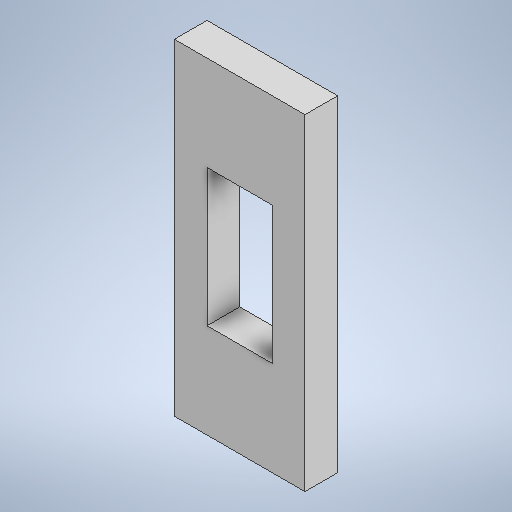
# Autodesk Inventor part: placa de amarre
Saved by Autodesk Inventor 2025.2 (Build 292293000, 293)
## iProperties
Created: 2025-03-06
Part Number: placa de amarre
Material: Genérico
Document SubType Name: Modeling
Designer: julia
Density: 1 g/cm^3
Appearance: Valor por defecto
Author: julia
Autodesk Inventor part; units mm, degrees
ref_plane "YZ Plane" through (0, 0, 0) normal (1, 0, 0) x (0, 1, 0)
ref_plane "XZ Plane" through (0, 0, 0) normal (0, 1, 0) x (-1, 0, 0)
ref_plane "XY Plane" through (0, 0, 0) normal (0, 0, 1) x (1, 0, 0)
sketch "Boceto1" plane through (0, 0, 0) normal (0, 0, 1) x (1, 0, 0)
  line L0 (0, 0) -> (2, 0)
  line L1 (2, 0) -> (2, 5)
  line L2 (2, 5) -> (0, 5)
  line L3 (0, 5) -> (0, 0)
  line L4 (0.5, 1.45) -> (1.5, 1.45)
  line L5 (1.5, 1.45) -> (1.5, 3.55)
  line L6 (1.5, 3.55) -> (0.5, 3.55)
  line L7 (0.5, 3.55) -> (0.5, 1.45)
  line L8 (0.5, 1.727) -> (0.5, 1.45)
  dimension "d0" = 2
  dimension "d1" = 5
  dimension "d2" = 1
  dimension "d3" = 2.1
  dimension "d5" = 1.45
  dimension "d6" = 0.5
  constraints: 18 end point, 4 parallel, 2 horizontal, 2 perpendicular
  measures "d0" distance of L2.end L1.end
  measures "d1" distance of L1.end L0.end
  measures "d2" distance of L6.end L5.end
  measures "d3" distance of L5.end L4.end
  measures "d5" distance from line of L0 L4.end
  measures "d6" distance from line of L3 L4.start
extrude "Extrusión1" add sketch "Boceto1" along normal blind 0.5
